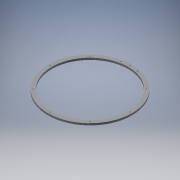
# Autodesk Inventor part: Base_Acryllic
Saved by Autodesk Inventor 2016 (Build 200138000, 138)
## iProperties
Created: 2016-03-29
Part Number: Base_Acryllic
Material: Generic
Document SubType Name: Modeling
Designer: Ethan
Density: 1 g/cm^3
Appearance: Default
Author: Ethan
Autodesk Inventor part; units mm, degrees
ref_plane "YZ Plane" through (0, 0, 0) normal (1, 0, 0) x (0, 1, 0)
ref_plane "XZ Plane" through (0, 0, 0) normal (0, 1, 0) x (-1, 0, 0)
ref_plane "XY Plane" through (0, 0, 0) normal (0, 0, 1) x (1, 0, 0)
sketch "Sketch1" plane through (0, 0, 0) normal (0, 1, 0) x (-1, 0, 0)
  arc A0 (42.8213, -132.9753) -> (-42.6787, -133.0211) centre (0, 0) ccw
  circle A1 centre (2.7003, 146.7014) radius 1.5875
  circle A2 centre (0, -133.35) radius 1.5875
  circle A3 centre (94.2927, -94.2927) radius 1.5875
  circle A4 centre (133.35, 0) radius 1.5875
  circle A5 centre (94.2927, 94.2927) radius 1.5875
  circle A6 centre (0, 133.35) radius 1.5875
  circle A7 centre (-94.2927, 94.2927) radius 1.5875
  circle A8 centre (-133.35, 0) radius 1.5875
  circle A9 centre (-94.2927, -94.2927) radius 1.5875
  arc A10 (42.8213, -119.5631) -> (-42.8213, -119.5631) centre (0, 0) ccw
  line L0 (1.5875, -133.35) -> (-1.5875, -133.35)
  arc A11 (-42.8213, -132.9753) -> (42.8213, -132.9753) centre (0, 0) ccw
  arc A12 (-42.8213, -119.5631) -> (42.8213, -119.5631) centre (0, 0) ccw
  circle A13 centre (-28.1555, -130.3624) radius 1.5875
  circle A14 centre (28.1555, -130.3624) radius 1.5875
  point P0 (-26.811, -129.5183)
  point P1 (-26.811, -129.5183)
  point P2 (26.811, -129.5183)
  point P3 (26.811, -129.5183)
  dimension "d97" = 3.175
  dimension "d134" = 3.175
  dimension "d135" = 133.35
  dimension "d138" = 360
  dimension "d140" = 254
  dimension "d157" = 3.175
  constraints: 15 centre point, 15 point on circle, 4 coincident, 2 end point, 1 concentric, 1 horizontal, 21 other
  measures "d97" diameter of A1
  measures "d134" diameter of A2
  measures "d135" distance of point (0, 0) A2.centre
  measures "d140" diameter of A10
  measures "d157" diameter of A13
extrude "Extrusion13" add sketch "Sketch1" along normal blind 6.35 contours A11 A0
body "Solid11"
